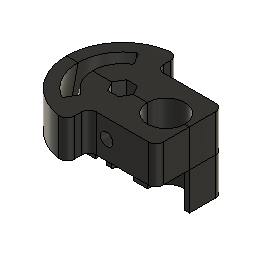
CableHolder (Autodesk Fusion 360 design; units mm, degrees)
Autodesk Fusion 360 part; units mm, degrees
sketch "Sketch1" plane through (0, 0, 12.7) normal (0, 0, 1) x (-1, 0, 0)
  circle A0 centre (0, -12.7) radius 3.031185
  circle A1 centre (0, -12.7) radius 2.0955
  line L0 (1.833087, -15.875) -> (3.666174, -12.7)
  line L1 (3.666174, -12.7) -> (1.833087, -9.525)
  line L2 (1.833087, -9.525) -> (-1.833087, -9.525)
  line L3 (-1.833087, -9.525) -> (-3.666174, -12.7)
  line L4 (-3.666174, -12.7) -> (-1.833087, -15.875)
  line L5 (-1.833087, -15.875) -> (1.833087, -15.875)
  line L6 (12.281684, -11.1125) -> (7.515657, -2.8575)
  line L7 (4.766026, -1.27) -> (-4.766026, -1.27)
  line L8 (-7.515657, -2.8575) -> (-12.281684, -11.1125)
  line L9 (-12.281684, -14.2875) -> (-7.515657, -22.5425)
  line L10 (-4.766026, -24.13) -> (4.766026, -24.13)
  line L11 (7.515657, -22.5425) -> (12.281684, -14.2875)
  arc A2 (4.766026, -24.13) -> (7.515657, -22.5425) centre (4.766026, -20.955) ccw
  arc A3 (-7.515657, -22.5425) -> (-4.766026, -24.13) centre (-4.766026, -20.955) ccw
  arc A4 (-12.281684, -11.1125) -> (-12.281684, -14.2875) centre (-9.532053, -12.7) ccw
  arc A5 (-4.766026, -1.27) -> (-7.515657, -2.8575) centre (-4.766026, -4.445) ccw
  arc A6 (7.515657, -2.8575) -> (4.766026, -1.27) centre (4.766026, -4.445) ccw
  arc A7 (12.281684, -14.2875) -> (12.281684, -11.1125) centre (9.532053, -12.7) ccw
  line L12 (12.707053, -12.7) -> (-12.707053, -12.7)
  line L13 (-10.167053, -24.13) -> (-4.766026, -24.13)
  arc A8 (-12.707053, -21.59) -> (-10.167053, -24.13) centre (-10.167053, -21.59) ccw
  line L14 (0, -25.505401) -> (-1.606531, -24.902736)
  line L15 (-12.707053, -21.59) -> (-12.707053, -12.7)
  line L16 (-12.707053, -22.245599) -> (-13.373578, -22.245599)
  line L17 (-9.532053, -12.7) -> (-22.867053, -12.7)
  line L18 (-4.766026, -24.13) -> (-22.867053, -24.13)
  line L19 (-25.407053, -21.59) -> (-25.407053, -15.24)
  arc A9 (-25.407053, -21.59) -> (-22.867053, -24.13) centre (-22.867053, -21.59) ccw
  arc A10 (-22.867053, -12.7) -> (-25.407053, -15.24) centre (-22.867053, -15.24) ccw
  line L20 (-12.707053, -12.7) -> (-3.666174, -12.7)
  line L21 (-8.186614, -12.7) -> (-4.150295, -12.7)
  line L22 (-4.150295, -12.7) -> (-25.407053, -12.7)
  circle A11 centre (-14.778674, -12.7) radius 6.35
  line L23 (-25.407053, -12.7) -> (-21.128674, -12.7)
  line L24 (-25.407053, -12.7) -> (-25.407053, -15.24)
  line L25 (-21.128674, -12.7) -> (-22.716174, -12.7)
  line L26 (-22.716174, -12.7) -> (-22.716174, -21.59)
  line L27 (-20.176174, -24.13) -> (-22.867053, -24.13)
  arc A12 (-22.716174, -21.59) -> (-20.176174, -24.13) centre (-20.176174, -21.59) ccw
  line L28 (-3.666174, -12.7) -> (-8.428674, -12.7)
  point P0 (0, -12.7)
  point P1 (-25.407053, -12.7)
  dimension "d1" = 3.175
  dimension "d3" = 3.175
  dimension "d38" = 2.54
  dimension "d115" = 15.875
  dimension "d116" = 2.54
  dimension "d118" = 12.7
  dimension "d119" = 1.5875
  dimension "d120" = 2.54
  dimension "d122" = 4.7625
  constraint coincident P0 A0.centre
  constraint tangent L10 A2
  constraint tangent L11 A2
  constraint tangent L9 A3
  constraint tangent L10 A3
  constraint equal A2 A3
  constraint tangent L8 A4
  constraint tangent L9 A4
  constraint equal A2 A4
  constraint tangent L7 A5
  constraint tangent L8 A5
  constraint equal A2 A5
  constraint tangent L6 A6
  constraint tangent L7 A6
  constraint equal A2 A6
  constraint tangent L6 A7
  constraint tangent L11 A7
  constraint equal A2 A7
  constraint horizontal L12
  constraint tangent A3 L13
  constraint tangent L13 A8
  constraint tangent A4 L15
  constraint perpendicular L15 L16
  constraint parallel L12 L17
  constraint tangent A3 L18
  constraint perpendicular L17 L19
  constraint tangent L18 A9
  constraint tangent L19 A9
  constraint tangent L17 A10
  constraint tangent L19 A10
  constraint equal A9 A10
  constraint perpendicular L15 L20
  constraint perpendicular L18 L26
  constraint tangent A9 L27
  constraint tangent L26 A12
  constraint tangent L27 A12
  constraint parallel L12 L28
  measures "d1" distance of P0 L5
  measures "d3" radius of A2
  measures "d38" radius of A8
  measures "d116" radius of A9
  measures "d118" diameter of A11
  measures "d120" radius of A12
extrude "Extrude1" add sketch "Sketch1" against normal blind 12.7 contours L0 L4 L5 L9 L10 L11 A2 A3 A7 L12 L20 L21 L22 A11 L28 | L9 A3 L13 A8 L15 L18 A11 | A8 L15 L17 L18 L22 A11 L23 L25 L26 A12 picked at (-0.611029, -21.378333) picked at (-10.463818, -20.685523) picked at (-16.104436, -21.69842) makes body 1
sketch "Sketch2" plane through (0, 12.7, 0) normal (0, -1, 0) x (1, 0, 0)
  line L0 (10.697, 12.7) -> (3.700693, 12.7)
  line L1 (3.700693, 12.7) -> (3.700693, 0)
  line L2 (3.700693, 0) -> (10.697, 0)
  line L3 (10.697, 0) -> (10.697, 12.7)
  circle A0 centre (6.047424, 6.35) radius 1.27
  line L4 (8.428674, 12.7) -> (3.666174, 12.7)
  line L5 (3.666174, 12.7) -> (3.666174, 0)
  line L6 (3.666174, 0) -> (8.428674, 0)
  line L7 (8.428674, 0) -> (8.428674, 12.7)
  dimension "d8" = 2.54
  measures "d8" diameter of A0
hole "Hole1" at (6.047424, 12.7, 6.35) direction (0, 1, 0) diameter 4.191 end up to surface (11.43 mm away) bodies 1
sketch "Sketch3" plane through (0, 0, 12.7) normal (0, 0, 1) x (-1, 0, 0)
  line L0 (3.666174, -12.7) -> (1.833087, -15.875)
  line L1 (1.833087, -15.875) -> (-1.833087, -15.875)
  line L2 (-1.833087, -15.875) -> (-3.666174, -12.7)
  line L3 (3.011078, 1.309549) -> (3.005466, 2.055514)
  line L4 (-3.666174, -12.7) -> (-8.428674, -12.7)
  line L5 (2.749631, -14.2875) -> (3.666174, -12.7)
  line L6 (3.207902, -13.49375) -> (3.124586, -13.435604)
  line L7 (4.538873, -12.7) -> (10.253873, -12.7)
  line L8 (3.526172, -14.6685) -> (6.415805, -14.6685) construction
  line L9 (4.090674, -12.7) -> (8.535674, -12.7)
  line L10 (3.779758, -14.2875) -> (12.379918, -14.2875) construction
  line L11 (3.526172, -14.6685) -> (7.408333, -14.6685) construction
  line L12 (9.89867, -18.415) -> (11.089705, -19.102644)
  line L13 (1.833087, -15.875) -> (2.056148, -16.010434)
  line L14 (-20.176174, -24.13) -> (4.766026, -24.13)
  arc A0 (4.766026, -24.13) -> (7.515657, -22.5425) centre (4.766026, -20.955) ccw
  line L15 (7.515657, -22.5425) -> (12.281684, -14.2875)
  arc A1 (12.281684, -14.2875) -> (12.707053, -12.7) centre (9.532053, -12.7) ccw
  line L16 (12.707053, -12.7) -> (3.666174, -12.7)
  ellipse E0 centre (0.278414, -12.919821) end of major axis (8.535674, -12.7) minor radius 7.923443 (7.375655, -16.958336) -> (7.375663, -16.958323) ccw
  ellipse E1 centre (0.278414, -12.919821) end of major axis (4.090674, -12.7) minor radius 3.509419 (-1.843546, -15.856884) -> (-1.813332, -15.875) ccw
  line L17 (2.749631, -14.2875) -> (9.89867, -18.415)
  line L18 (6.324151, -16.35125) -> (8.432201, -12.7)
  line L19 (6.324151, -16.35125) -> (10.540251, -16.35125) construction
  circle A2 centre (7.295687, -14.6685) radius 1.9685
  line L20 (7.295687, -14.6685) -> (7.295687, -12.7)
  line L21 (5.327187, -14.6685) -> (5.327187, -12.7)
  line L22 (9.264187, -12.7) -> (9.264187, -16.152412)
  line L23 (-21.128674, -12.7) -> (-22.716174, -12.7)
  arc A3 (-21.128674, -12.7) -> (-8.428674, -12.7) centre (-14.778674, -12.7) ccw
  line L24 (-22.716174, -12.7) -> (-22.716174, -21.59)
  arc A4 (-22.716174, -21.59) -> (-20.176174, -24.13) centre (-20.176174, -21.59) ccw
  dimension "d32" = 0.1016
  dimension "d41" = 4.445
  dimension "d76" = 60
  dimension "d77" = 3.937
  dimension "d78" = 1.9685
  constraint horizontal L8
  constraint horizontal L10
  constraint horizontal L11
  constraint perpendicular L15 L17
  constraint horizontal L19
  constraint perpendicular L10 L20
  constraint vertical L21
  constraint tangent A2 L21
  constraint perpendicular L10 L22
  constraint tangent A2 L22
  measures "d76" angle of L18 L19
  measures "d77" diameter of A2
extrude "Extrude6" cut sketch "Sketch3" against normal blind 12.7 contours L17 L18 A2 L20 | L17 A2 | L7 L9 L16 A2 L21 | L1 L2 E1 | L17 L18 A2 | L7 L9 L16 L18 A2 | L18 A2 L20 | L7 L9 L16 L18 A2 L22 picked at (6.556955, -15.73777) picked at (6.441889, -16.427924) picked at (5.713925, -13.086738) picked at (-1.827485, -15.87049) picked at (6.739037, -15.842896) picked at (8.253712, -12.837857) picked at (7.381334, -13.36178) picked at (8.774296, -12.843155) bodies 1
move_body "Move1" bodies 1 to x (1, 0, 0) y (0, 1, 0) z (0, 0, 1) at (0, 0, -12.7)
sketch "Sketch7" plane through (0, 0, 12.7) normal (0, 0, 1) x (-1, 0, 0)
  circle A0 centre (0, -12.7) radius 3.031185
  circle A1 centre (0, -12.7) radius 2.0955
  line L0 (-1.833087, -9.525) -> (-3.666174, -12.7)
  line L1 (-3.666174, -12.7) -> (-1.833087, -15.875)
  line L2 (-1.833087, -15.875) -> (1.833087, -15.875)
  line L3 (1.833087, -15.875) -> (3.666174, -12.7)
  line L4 (3.666174, -12.7) -> (1.833087, -9.525)
  line L5 (1.833087, -9.525) -> (-1.833087, -9.525)
  line L6 (0, -32.385) -> (0, -26.67)
  line L7 (-2.54, -24.13) -> (-10.29161, -24.13)
  line L8 (-12.707053, -21.714556) -> (-12.707053, -12.7)
  arc A2 (0, -26.67) -> (-2.54, -24.13) centre (-2.54, -26.67) ccw
  arc A3 (-12.707053, -21.714556) -> (-10.29161, -24.13) centre (-10.29161, -21.714556) ccw
  circle A4 centre (0, -12.7) radius 19.05
  line L9 (-12.707053, -12.7) -> (19.05, -12.7)
  line L10 (-3.666174, -12.7) -> (-8.428674, -12.7)
  circle A5 centre (-14.778674, -12.7) radius 6.35
  line L11 (-21.128674, -12.7) -> (-22.716174, -12.7)
  line L12 (-22.716174, -12.7) -> (-22.716174, -21.59)
  line L13 (-20.176174, -24.13) -> (-10.29161, -24.13)
  arc A6 (-22.716174, -21.59) -> (-20.176174, -24.13) centre (-20.176174, -21.59) ccw
  point P0 (0, -12.7)
  point P1 (0, -34.925)
  point P2 (0, -24.13)
  dimension "d79" = 3.175
  dimension "d82" = 10.795
  dimension "d91" = 38.1
  dimension "d124" = 4.7625
  dimension "d125" = 12.7
  dimension "d126" = 1.5875
  dimension "d127" = 2.54
  constraint coincident P0 A0.centre
  constraint coincident P1 L6
  constraint coincident P2 L6
  constraint coincident P2 L7
  constraint tangent L6 A2
  constraint tangent L7 A2
  constraint tangent L7 A3
  constraint tangent L8 A3
  constraint coincident A4 L9.end
  constraint parallel L9 L10
  constraint parallel L9 L11
  constraint perpendicular L7 L12
  constraint tangent A3 L13
  constraint tangent L12 A6
  constraint tangent L13 A6
  measures "d79" distance of P0 L5
  measures "d82" distance of P1 P2
  measures "d91" diameter of A4
  measures "d125" diameter of A5
  measures "d127" radius of A6
extrude "Extrude8" add sketch "Sketch7" along normal blind 12.7 separate body contours L1 L2 L3 L6 L7 L8 A2 A3 A4 L9 L10 A5 | L8 A3 A4 A5 L13 | A4 A5 L11 L12 L13 A6 picked at (3.967587, -23.405242) picked at (-14.517675, -20.986249) picked at (-20.141706, -21.95671) makes body 2
sketch "Sketch8" plane through (0, 12.7, 0) normal (0, -1, 0) x (1, 0, 0)
  line L0 (3.666174, 12.7) -> (8.428674, 12.7)
  line L1 (8.428674, 25.4) -> (3.666174, 25.4)
  line L2 (3.666174, 25.4) -> (3.666174, 12.7)
  circle A0 centre (6.002974, 19.05) radius 1.27
  line L3 (8.428674, 12.7) -> (8.428674, 25.4)
  line L4 (6.002974, 19.05) -> (3.666174, 19.05)
  dimension "d86" = 2.54
  dimension "d141" = 2.3368
  constraint perpendicular L2 L4
  measures "d86" diameter of A0
hole "Hole4" at (6.002974, 12.7, 19.05) direction (0, 1, 0) diameter 4.191 end up to surface (11.43 mm away) bodies 2
fillet "Fillet7" radius 2.54 1 edges at (0, 31.75, 19.05) on bodies 2
move_body "Move2" bodies 2 to x (1, 0, 0) y (0, 1, 0) z (0, 0, 1) at (0, 0, -12.7)
sketch "Sketch12" plane through (0, 12.7, 0) normal (0, -1, 0) x (1, 0, 0)
  line L0 (-19.05, 0) -> (-3.666174, 0)
  line L1 (-3.666174, 0) -> (-3.666174, 12.7)
  line L2 (-3.666174, 12.7) -> (-19.05, 12.7)
  line L3 (-19.05, 12.7) -> (-19.05, 0)
  line L4 (-3.666174, 0) -> (-12.70705, 0)
  line L5 (-12.70705, 0) -> (-17.46955, 0)
  line L6 (-17.46955, 0) -> (-15.0883, 0)
  line L7 (-15.0883, 0) -> (-15.0883, 12.7)
  line L8 (-17.46955, 0) -> (-15.0883, 12.7)
  line L9 (-16.278925, 6.35) -> (-11.597996, 5.472326)
  line L10 (-11.597996, 5.472326) -> (-12.70705, 0)
  line L11 (-11.597996, 5.472326) -> (-10.242808, 12.7)
  line L12 (-15.0883, 12.7) -> (-10.242808, 12.7)
  dimension "d128" = 9.040876
  dimension "d129" = 4.7625
  dimension "d131" = 4.7625
  constraint perpendicular L3 L5
  constraint midpoint L5 L6.end
  constraint coincident L2 L7.end
  constraint perpendicular L2 L7
  constraint perpendicular L8 L9
  constraint perpendicular L9 L11
sketch "Sketch13" plane through (0, 0, 12.7) normal (0, 0, 1) x (-1, 0, 0)
  arc A0 (0, -29.013445) -> (2.930769, -31.523206) centre (2.54, -29.013445) ccw
  arc A1 (2.930769, -31.523206) -> (19.05, -12.7) centre (0, -12.7) ccw
  line L0 (19.05, -12.7) -> (3.666174, -12.7)
  line L1 (3.666174, -12.7) -> (1.833087, -15.875)
  line L2 (1.833087, -15.875) -> (-1.833087, -15.875)
  line L3 (-1.833087, -15.875) -> (-3.666174, -12.7)
  line L4 (-3.666174, -12.7) -> (-8.428674, -12.7)
  arc A2 (-21.128674, -12.7) -> (-8.428674, -12.7) centre (-14.778674, -12.7) ccw
  line L5 (-21.128674, -12.7) -> (-22.716174, -12.7)
  line L6 (-22.716174, -12.7) -> (-22.716174, -21.59)
  arc A3 (-22.716174, -21.59) -> (-20.176174, -24.13) centre (-20.176174, -21.59) ccw
  line L7 (-20.176174, -24.13) -> (-2.54, -24.13)
  arc A4 (0, -26.67) -> (-2.54, -24.13) centre (-2.54, -26.67) ccw
  line L8 (0, -26.67) -> (0, -29.013445)
  circle A5 centre (0, -12.7) radius 1.27
  dimension "d132" = 2.54
  constraint concentric A1 A5
  measures "d132" diameter of A5
copy_body "CopyPasteBodies1" bodies 2 makes body 3
move_body "Move3" bodies 3 to x (1, 0, 0) y (0, -1, 0) z (0, 0, -1) at (0, 25.4, 12.7)
revolve "Revolve1" cut sketch "Sketch12" angle 60 about axis through (0, 12.7, 11.43) along (0, 0, -1) contours L0 L5 L6 L7 L8 L9 | L0 L5 L7 L9 L10 | L7 L8 L9 | L2 L7 L9 L11 L12 picked at (-15.88205, 2.042252) picked at (-13.131116, 3.866361) picked at (-15.485175, 8.392252) picked at (-12.309701, 10.290775) bodies 2
fillet "Fillet8" radius 0.635 3 edges at (-8.139463, 26.797963, 6.35) (-5.460201, 22.157345, 9.086163) (-6.076262, 23.224394, 2.736163) on bodies 2
revolve "Revolve2" cut sketch "Sketch12" angle 60 about axis through (0, 12.7, 11.43) along (0, 0, 1) contours L0 L5 L6 L7 L8 L9 | L0 L5 L7 L9 L10 | L7 L8 L9 | L2 L7 L9 L11 L12 picked at (-15.88205, 2.042252) picked at (-13.131116, 3.866361) picked at (-15.485175, 8.392252) picked at (-12.309701, 10.290775) bodies 3
fillet "Fillet9" radius 0.635 3 edges at (-5.460201, 3.242654, 9.086163) (-6.076262, 2.175606, 2.736163) (-8.139463, -1.397963, 6.35) on bodies 3
equation "d4 = ( -1 / 2 ) * 1 in"
equation "d78 = ( 0.155 / 2 ) * 1 in"
equation "d119 = ( 1 / 16 ) * 1 in"
equation "d126 = ( 1 / 16 ) * 1 in"
named bodies: "CableHolderClose", "CableHolderFar", "CableHolderFar2"
